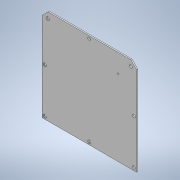
# Autodesk Inventor part: tampa da caixa de engrenagem
Saved by Autodesk Inventor 2022.1 (Build 261234020, 234B)
## iProperties
Created: 2023-10-20
Part Number: tampa da caixa de engrenagem
Material: Generic
Document SubType Name: Modeling
Designer: SENAI
Density: 1 g/cm^3
Appearance: Default
Author: SENAI
Autodesk Inventor part; units mm, degrees
ref_plane "YZ Plane" through (0, 0, 0) normal (1, 0, 0) x (0, 1, 0)
ref_plane "XZ Plane" through (0, 0, 0) normal (0, 1, 0) x (-1, 0, 0)
ref_plane "XY Plane" through (0, 0, 0) normal (0, 0, 1) x (1, 0, 0)
sketch "Sketch1" plane through (0, 0, 0) normal (0, 0, 1) x (1, 0, 0)
  line L0 (230, 0) -> (0, 0)
  line L1 (14.5, 230) -> (215.5, 230)
  line L2 (0, 215.5) -> (0, 0)
  line L3 (0, 215.5) -> (14.5, 230)
  line L4 (230, 215.5) -> (230, 0)
  line L5 (215.5, 230) -> (230, 215.5)
  dimension "d6" = 135
  dimension "d7" = 230
  dimension "d8" = 230
  dimension "d9" = 315.0161
  dimension "d10" = 152.3815
  constraints: 12 end point, 2 perpendicular, 1 horizontal, 1 parallel, 1 vertical
  measures "d6" angle of L4 L5
  measures "d7" distance between parallel lines of L4 L2
  measures "d8" distance between parallel lines of L1 L0
  measures "d9" distance from line of L0.end L5
  measures "d10" distance from line of L0.end L3
extrude "Extrusion1" add sketch "Sketch1" along normal blind 3
sketch "Sketch2" plane through (0, 0, 3) normal (0, 0, 1) x (1, 0, 0)
  line L0 (215.5, 230) -> (14.5, 230) projected
  circle A0 centre (115, 223.25) radius 3.75
  line L1 (0, 0) -> (230, 0) projected
  circle A1 centre (115, 6.75) radius 3.75
  line L2 (0, 215.5) -> (0, 0) projected
  circle A2 centre (6.75, 115) radius 3.75
  line L3 (230, 0) -> (230, 215.5) projected
  circle A3 centre (223.25, 115) radius 3.75
  circle A4 centre (6.75, 6.75) radius 3.75
  circle A5 centre (223.25, 6.75) radius 3.75
  line L4 (14.5, 230) -> (0, 215.5) projected
  circle A6 centre (14.1443, 215.8557) radius 3.75
  line L5 (230, 215.5) -> (215.5, 230) projected
  circle A7 centre (215.8557, 215.8557) radius 3.75
  circle A8 centre (185, 185) radius 1.5
  dimension "d19" = 7.5
  dimension "d21" = 7.5
  dimension "d23" = 7.5
  dimension "d25" = 7.5
  dimension "d28" = 7.5
  dimension "d31" = 7.5
  dimension "d34" = 7.5
  dimension "d37" = 7.5
  dimension "d43" = 3
  constraints: 9 centre point
  measures "d19" diameter of A0
  measures "d21" diameter of A1
  measures "d23" diameter of A2
  measures "d25" diameter of A3
  measures "d28" diameter of A4
  measures "d31" diameter of A5
  measures "d34" diameter of A6
  measures "d37" diameter of A7
  measures "d43" diameter of A8
extrude "Extrusion2" cut sketch "Sketch2" against normal through all contours A0 | A1 | A2 | A3 | A4 | A5 | A6 | A7 | A8
body "Solid1"
